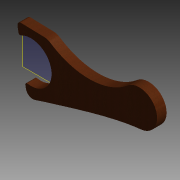
# Autodesk Inventor part: body01
Saved by Autodesk Inventor 2013 (Build 170138000, 138)
## iProperties
Created: 2013-02-19
Part Number: body01
Material: Wood (Walnut)
Document SubType Name: Modeling
Designer: Nano
Density: 0.55 g/cm^3
Mass: 9079.15 g
Surface Area: 6785.14 cm^2
Volume: 16507.6 cm^3
Author: Nano
Autodesk Inventor part; units mm, degrees
ref_plane "YZ Plane" through (0, 0, 0) normal (1, 0, 0) x (0, 1, 0)
ref_plane "XZ Plane" through (0, 0, 0) normal (0, 1, 0) x (-1, 0, 0)
ref_plane "XY Plane" through (0, 0, 0) normal (0, 0, 1) x (1, 0, 0)
ref_plane "Work Plane1" through (0, 0, -22.225) normal (0, 0, -1) x (-1, 0, 0)
sketch "Sketch1" plane through (0, 0, -22.225) normal (0, 0, -1) x (-1, 0, 0)
  arc A0 (88.9626, 123.799) -> (43.8693, -146.1511) centre (0.2092, -0.1167) ccw
  line L0 (104.0584, 214.2592) -> (-123.3104, 207.8545)
  line L1 (104.0584, 214.2592) -> (88.9626, 123.799)
  line L2 (27.3448, -245.173) -> (43.8693, -146.1511)
  spline S0 degree 3 poles (-707.521, 203.2816) (-551.4111, 75.786) (-311.6058, 71.5174) (-123.3104, 207.8545) knots 0 0 0 0 1 1 1 1
  spline S1 degree 3 poles (-813.9039, -23.98) (-592.8487, -45.4285) (-280.1393, -149.9031) (-98.6304, -203.95) knots 0 0 0 0 1 1 1 1
  line L3 (-98.6304, -203.95) -> (27.3448, -245.173)
  arc A1 (-707.521, 203.2816) -> (-707.521, 203.2816) centre (-797.0248, 106.6489) ccw
  arc A2 (-707.521, 203.2816) -> (-707.521, 203.2816) centre (-797.0248, 106.6489) ccw
  line L4 (-754.135, 241.3513) -> (-660.9071, 165.2118) construction
  arc A3 (-742.7917, 235.6937) -> (-668.7166, 175.1963) centre (-447.712, 521.4005) ccw construction
  line L5 (-880.3002, -17.5377) -> (-747.5076, -30.4223) construction
  arc A4 (-760.9988, -30.537) -> (-867.0828, -20.2439) centre (-910.7419, -1022.0239) ccw construction
  arc A5 (-707.521, 203.2816) -> (-807.2552, -24.6472) centre (-797.0248, 106.6609) ccw
  point P0 (-439.0779, 106.766)
  point P1 (-428.475, -105.3455)
  constraints: 13 end point, 6 point on circle, 4 centre point, 4 midpoint, 24 other
extrude "Extrusion1" add sketch "Sketch1" against normal blind 69.85 contours A0 L2 L3 S1 A1 S0 L0 L1 | A1 S1 A5 | A1 A5 | A5 S1 A1 | A5 S1 picked at (-813.5215, 64.1011) picked at (-885.4144, 33.6038)
fillet "Fillet1" radius 25.4 1 edges at (-104.0584, 214.2592, 12.7)
fillet "Fillet2" radius 50.8 1 edges at (-27.3448, -245.173, 12.7)
fillet "Fillet4" radius 76.2 1 edges at (123.3104, 207.8545, 12.7)
fillet "Fillet5" radius 12.7 2 edges at (-43.8693, -146.1511, 12.7) (-88.9626, 123.799, 12.7)
body "Solid1"
